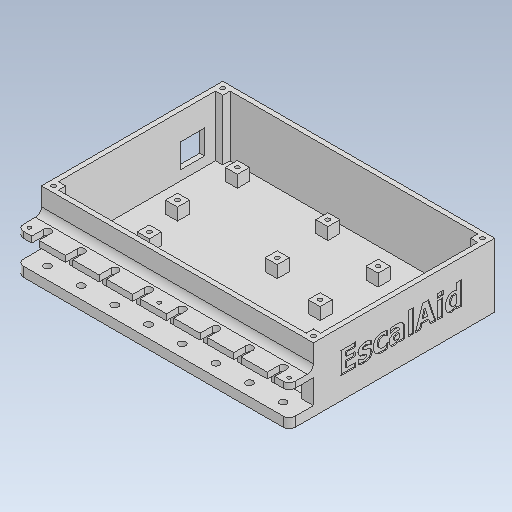
# Autodesk Inventor part: ebox
Saved by Autodesk Inventor 2025.2 (Build 292293000, 293)
## iProperties
Created: 2025-01-01
Part Number: ebox
Material: Generic
Document SubType Name: Modeling
Designer: email
Density: 1 g/cm^3
Appearance: Default
Author: email
Autodesk Inventor part; units mm, degrees
ref_plane "YZ Plane" through (0, 0, 0) normal (1, 0, 0) x (0, 1, 0)
ref_plane "XZ Plane" through (0, 0, 0) normal (0, 1, 0) x (-1, 0, 0)
sketch "Sketch1" plane through (0, 0, 0) normal (0, 1, 0) x (-1, 0, 0)
  line L0 (0, 0) -> (-225, 0)
  line L1 (-225, 0) -> (-225, -150)
  line L2 (-225, -150) -> (0, -150)
  line L3 (0, -150) -> (0, 0)
  line L4 (-12.5, -136.845) -> (-114.1, -136.845)
  line L5 (-114.1, -136.845) -> (-114.1, -83.505)
  line L6 (-114.1, -83.505) -> (-12.5, -83.505)
  line L7 (-12.5, -83.505) -> (-12.5, -136.845)
  line L8 (-4, -4) -> (-221, -4)
  line L9 (-221, -4) -> (-221, -146)
  line L10 (-221, -146) -> (-4, -146)
  line L11 (-4, -146) -> (-4, -4)
  line L12 (-153.3391, -125.2346) -> (-208.3391, -125.2346)
  line L13 (-208.3391, -125.2346) -> (-208.3391, -70.2346)
  line L14 (-208.3391, -70.2346) -> (-153.3391, -70.2346)
  line L15 (-153.3391, -70.2346) -> (-153.3391, -125.2346)
  line L16 (-12.6469, -54.1694) -> (-42.6469, -54.1694)
  line L17 (-42.6469, -54.1694) -> (-42.6469, -34.1694)
  line L18 (-42.6469, -34.1694) -> (-12.6469, -34.1694)
  line L19 (-12.6469, -34.1694) -> (-12.6469, -54.1694)
  line L20 (-15.41, -128.945) -> (-4, -128.945)
  line L21 (-4, -128.945) -> (-4, -117.045)
  line L22 (-4, -117.045) -> (-15.41, -117.045)
  line L23 (-15.41, -117.045) -> (-15.41, -128.945)
  circle A0 centre (-27.74, -134.305) radius 1.75
  circle A1 centre (-26.47, -86.045) radius 1.75
  circle A2 centre (-102.67, -134.305) radius 1.75
  circle A3 centre (-109.02, -86.045) radius 1.75
  circle A4 centre (-156.8391, -121.7346) radius 1.75
  circle A5 centre (-204.8391, -121.7346) radius 1.75
  circle A6 centre (-156.8391, -73.7346) radius 1.75
  circle A7 centre (-204.8391, -73.7346) radius 1.75
  circle A8 centre (-37.5669, -51.6294) radius 1.75
  circle A9 centre (-37.5669, -36.7094) radius 1.75
  line L24 (-22.74, -139.305) -> (-32.74, -139.305)
  line L25 (-32.74, -139.305) -> (-32.74, -129.305)
  line L26 (-32.74, -129.305) -> (-22.74, -129.305)
  line L27 (-22.74, -129.305) -> (-22.74, -139.305)
  line L28 (-22.74, -139.305) -> (-32.74, -129.305) construction
  line L29 (-32.74, -139.305) -> (-22.74, -129.305) construction
  line L30 (-21.47, -81.045) -> (-31.47, -81.045)
  line L31 (-31.47, -81.045) -> (-31.47, -91.045)
  line L32 (-31.47, -91.045) -> (-21.47, -91.045)
  line L33 (-21.47, -91.045) -> (-21.47, -81.045)
  line L34 (-21.47, -81.045) -> (-31.47, -91.045) construction
  line L35 (-31.47, -81.045) -> (-21.47, -91.045) construction
  line L36 (-114.02, -81.045) -> (-104.02, -81.045)
  line L37 (-104.02, -81.045) -> (-104.02, -91.045)
  line L38 (-104.02, -91.045) -> (-114.02, -91.045)
  line L39 (-114.02, -91.045) -> (-114.02, -81.045)
  line L40 (-114.02, -81.045) -> (-104.02, -91.045) construction
  line L41 (-104.02, -81.045) -> (-114.02, -91.045) construction
  line L42 (-107.67, -139.305) -> (-97.67, -139.305)
  line L43 (-97.67, -139.305) -> (-97.67, -129.305)
  line L44 (-97.67, -129.305) -> (-107.67, -129.305)
  line L45 (-107.67, -129.305) -> (-107.67, -139.305)
  line L46 (-107.67, -139.305) -> (-97.67, -129.305) construction
  line L47 (-97.67, -139.305) -> (-107.67, -129.305) construction
  line L48 (-151.8391, -126.7346) -> (-161.8391, -126.7346)
  line L49 (-161.8391, -126.7346) -> (-161.8391, -116.7346)
  line L50 (-161.8391, -116.7346) -> (-151.8391, -116.7346)
  line L51 (-151.8391, -116.7346) -> (-151.8391, -126.7346)
  line L52 (-151.8391, -126.7346) -> (-161.8391, -116.7346) construction
  line L53 (-161.8391, -126.7346) -> (-151.8391, -116.7346) construction
  line L54 (-209.8391, -126.7346) -> (-199.8391, -126.7346)
  line L55 (-199.8391, -126.7346) -> (-199.8391, -116.7346)
  line L56 (-199.8391, -116.7346) -> (-209.8391, -116.7346)
  line L57 (-209.8391, -116.7346) -> (-209.8391, -126.7346)
  line L58 (-209.8391, -126.7346) -> (-199.8391, -116.7346) construction
  line L59 (-199.8391, -126.7346) -> (-209.8391, -116.7346) construction
  line L60 (-209.8391, -68.7346) -> (-199.8391, -68.7346)
  line L61 (-199.8391, -68.7346) -> (-199.8391, -78.7346)
  line L62 (-199.8391, -78.7346) -> (-209.8391, -78.7346)
  line L63 (-209.8391, -78.7346) -> (-209.8391, -68.7346)
  line L64 (-209.8391, -68.7346) -> (-199.8391, -78.7346) construction
  line L65 (-199.8391, -68.7346) -> (-209.8391, -78.7346) construction
  line L66 (-161.8391, -68.7346) -> (-151.8391, -68.7346)
  line L67 (-151.8391, -68.7346) -> (-151.8391, -78.7346)
  line L68 (-151.8391, -78.7346) -> (-161.8391, -78.7346)
  line L69 (-161.8391, -78.7346) -> (-161.8391, -68.7346)
  line L70 (-161.8391, -68.7346) -> (-151.8391, -78.7346) construction
  line L71 (-151.8391, -68.7346) -> (-161.8391, -78.7346) construction
  line L72 (-42.5669, -46.6294) -> (-32.5669, -46.6294)
  line L73 (-32.5669, -46.6294) -> (-32.5669, -56.6294)
  line L74 (-32.5669, -56.6294) -> (-42.5669, -56.6294)
  line L75 (-42.5669, -56.6294) -> (-42.5669, -46.6294)
  line L76 (-42.5669, -46.6294) -> (-32.5669, -56.6294) construction
  line L77 (-32.5669, -46.6294) -> (-42.5669, -56.6294) construction
  line L78 (-32.5669, -41.7094) -> (-42.5669, -41.7094)
  line L79 (-42.5669, -41.7094) -> (-42.5669, -31.7094)
  line L80 (-42.5669, -31.7094) -> (-32.5669, -31.7094)
  line L81 (-32.5669, -31.7094) -> (-32.5669, -41.7094)
  line L82 (-32.5669, -41.7094) -> (-42.5669, -31.7094) construction
  line L83 (-42.5669, -41.7094) -> (-32.5669, -31.7094) construction
  line L84 (0, -4) -> (-225, -4)
  line L85 (-225, -4) -> (-225, 20)
  line L86 (-225, 20) -> (0, 20)
  line L87 (0, 20) -> (0, -4)
  circle A10 centre (-15, 10) radius 2.95
  circle A11 centre (-42.85, 10) radius 2.95
  circle A12 centre (-70.7, 10) radius 2.95
  circle A13 centre (-98.55, 10) radius 2.95
  circle A14 centre (-126.4, 10) radius 2.95
  circle A15 centre (-154.25, 10) radius 2.95
  circle A16 centre (-182.1, 10) radius 2.95
  circle A17 centre (-209.95, 10) radius 2.95
  point P0 (-156.8391, -73.7346)
  point P1 (-225, 8)
  dimension "d0" = 225
  dimension "d1" = 150
  dimension "d2" = 101.6
  dimension "d3" = 53.34
  dimension "d5" = 4
  dimension "d6" = 217
  dimension "d7" = 142
  dimension "d8" = 4
  dimension "d9" = 8.5
  dimension "d10" = 55
  dimension "d11" = 55
  dimension "d12" = 30
  dimension "d13" = 20
  dimension "d14" = 7.9
  dimension "d15" = 8.5
  dimension "d16" = 11.9
  dimension "d17" = 2.54
  dimension "d18" = 3.5
  dimension "d19" = 15.24
  dimension "d20" = 3.5
  dimension "d21" = 3.5
  dimension "d22" = 3.5
  dimension "d23" = 2.54
  dimension "d24" = 13.97
  dimension "d26" = 2.54
  dimension "d27" = 90.17
  dimension "d28" = 2.54
  dimension "d29" = 96.52
  dimension "d30" = 3.5
  dimension "d31" = 3.5
  dimension "d32" = 3.5
  dimension "d33" = 3.5
  dimension "d34" = 3.5
  dimension "d35" = 3.5
  dimension "d36" = 3.5
  dimension "d38" = 3.5
  dimension "d39" = 3.5
  dimension "d40" = 3.5
  dimension "d41" = 3.5
  dimension "d42" = 3.5
  dimension "d43" = 3.5
  dimension "d44" = 2.54
  dimension "d45" = 5.08
  dimension "d46" = 5.08
  dimension "d47" = 2.54
  dimension "d54" = 10
  dimension "d55" = 10
  dimension "d56" = 10
  dimension "d57" = 10
  dimension "d58" = 10
  dimension "d59" = 10
  dimension "d60" = 10
  dimension "d61" = 10
  dimension "d65" = 10
  dimension "d66" = 10
  dimension "d67" = 10
  dimension "d68" = 10
  dimension "d69" = 10
  dimension "d70" = 10
  dimension "d71" = 10
  dimension "d72" = 10
  dimension "d73" = 10
  dimension "d74" = 10
  dimension "d75" = 10
  constraints: 176 end point, 34 parallel, 22 midpoint, 18 centre point, 18 horizontal, 17 perpendicular, 2 point on line, 14 other
  measures "d0" distance of L1.end L2.end
  measures "d1" distance of L0.end L1.end
  measures "d2" distance of L4.start L4.end
  measures "d3" distance of L4.end L5.end
  measures "d5" distance between parallel lines of L0 L8
  measures "d6" distance of L9.end L10.end
  measures "d7" distance of L8.end L9.end
  measures "d8" distance between parallel lines of L3 L11
  measures "d9" distance between parallel lines of L11 L7
  measures "d10" distance of L12.end L13.end
  measures "d11" distance of L13.end L14.end
  measures "d12" distance of L16.start L16.end
  measures "d13" distance of L16.end L17.end
  measures "d14" distance between parallel lines of L4 L20
  measures "d15" distance between parallel lines of L7 L21
  measures "d16" distance of L22.end L20.start
  measures "d17" distance from line of L4 A0.centre
  measures "d18" diameter of A0
  measures "d19" distance from line of L7 A0.centre
  measures "d20" diameter of A1
  measures "d21" diameter of A3
  measures "d22" diameter of A2
  measures "d23" distance from line of L6 A1.centre
  measures "d24" distance from line of L7 A1.centre
  measures "d26" distance from line of L4 A2.centre
  measures "d27" distance from line of A2.centre L7
  measures "d28" distance from line of L6 A3.centre
  measures "d29" distance from line of L7 A3.centre
  measures "d30" diameter of A4
  measures "d31" diameter of A5
  measures "d32" diameter of A6
  measures "d33" diameter of A7
  measures "d34" distance from line of L12 A4.centre
  measures "d35" distance from line of L15 A4.centre
  measures "d36" distance from line of L14 A6.centre
  measures "d38" distance from line of L13 A7.centre
  measures "d39" distance from line of L14 A7.centre
  measures "d40" distance from line of L13 A5.centre
  measures "d41" distance from line of L12 A5.centre
  measures "d42" diameter of A8
  measures "d43" diameter of A9
  measures "d44" distance from line of L16 A8.centre
  measures "d45" distance from line of L17 A8.centre
  measures "d46" distance from line of L17 A9.centre
  measures "d47" distance from line of L18 A9.centre
  measures "d54" distance of L24.end L25.end
  measures "d55" distance of L25.end L26.end
  measures "d56" distance of L42.end L43.end
  measures "d57" distance of L43.end L44.end
  measures "d58" distance of L31.end L32.end
  measures "d59" distance of L30.end L31.end
  measures "d60" distance of L37.end L38.end
  measures "d61" distance of L36.end L37.end
  measures "d65" distance of L48.end L49.end
  measures "d66" distance of L49.end L50.end
  measures "d67" distance of L54.end L55.end
  measures "d68" distance of L55.end L56.end
  measures "d69" distance of L66.end L67.end
  measures "d70" distance of L66.start L66.end
  measures "d71" distance of L62.end L60.start
  measures "d72" distance of L60.start L60.end
  measures "d73" distance of L73.end L74.end
  measures "d74" distance of L72.end L73.end
  measures "d75" distance of L78.start L78.end
extrude "Extrusion1" add sketch "Sketch1" against normal blind 3 contours L3 L84 L8 L1 L0 | L3 L2 L1 L84 L9 L10 L11 | L11 L22 L7 L6 L33 L30 L31 L37 L36 L39 L5 L4 L45 L42 L43 L25 L24 L27 L20 L10 L9 L8 | L11 L20 L7 L22 | L22 L23 L20 L7 L4 L27 L26 L25 L43 L44 L45 L5 L6 L39 L38 L37 L31 L32 L33 | L7 L20 L23 L22 | L33 L32 L31 L6 | L6 L31 L30 L33 | L27 L24 L25 L4 | L4 L25 L26 L27 | L37 L38 L39 L6 | L6 L39 L36 L37 | L43 L42 L45 L4 | L4 L45 L44 L43 | L15 L50 L51 L48 L49 L12 | L12 L49 L50 L15 | L12 L55 L56 L13 L62 L61 L14 L69 L68 L15 L50 L49 | L55 L54 L57 L56 L13 L12 | L12 L13 L56 L55 | L68 L69 L14 L15 | L15 L14 L69 L66 L67 L68 | L62 L63 L60 L61 L14 L13 | L13 L14 L61 L62 | L16 L73 L72 L75 L17 L18 L79 L78 L81 L19 | L73 L74 L75 L16 | L16 L75 L72 L73 | L81 L78 L79 L18 | L18 L79 L80 L81 | A0 | A1 | A2 | A3 | A4 | A5 | A6 | A7 | A8 | A9
extrude "Extrusion2" add sketch "Sketch1" along normal blind 50 contours L3 L84 L8 L1 L0 | L3 L2 L1 L84 L9 L10 L11
extrude "Extrusion3" add sketch "Sketch1" along normal blind 10 contours L33 L32 L31 L6 | L6 L31 L30 L33 | L27 L24 L25 L4 | L4 L25 L26 L27 | L37 L38 L39 L6 | L6 L39 L36 L37 | L43 L42 L45 L4 | L4 L45 L44 L43 | L15 L50 L51 L48 L49 L12 | L12 L49 L50 L15 | L55 L54 L57 L56 L13 L12 | L12 L13 L56 L55 | L68 L69 L14 L15 | L15 L14 L69 L66 L67 L68 | L62 L63 L60 L61 L14 L13 | L13 L14 L61 L62 | L73 L74 L75 L16 | L16 L75 L72 L73 | L81 L78 L79 L18 | L18 L79 L80 L81
extrude "Extrusion4" add sketch "Sketch1" along normal blind 5 and the other way blind 3 contours L0 L85 L86 L87
sketch "Sketch2" plane through (0, 50, 0) normal (0, 0, 1) x (1, 0, 0)
  line L0 (7, -25) -> (23, -25)
  line L1 (23, -25) -> (23, -45)
  line L2 (23, -45) -> (7, -45)
  line L3 (7, -45) -> (7, -25)
  line L4 (7, -25) -> (23, -45) construction
  line L5 (23, -25) -> (7, -45) construction
  line L6 (34.85, -25) -> (50.85, -25)
  line L7 (50.85, -25) -> (50.85, -45)
  line L8 (50.85, -45) -> (34.85, -45)
  line L9 (34.85, -45) -> (34.85, -25)
  line L10 (34.85, -25) -> (50.85, -45) construction
  line L11 (50.85, -25) -> (34.85, -45) construction
  line L12 (62.7, -25) -> (78.7, -25)
  line L13 (78.7, -25) -> (78.7, -45)
  line L14 (78.7, -45) -> (62.7, -45)
  line L15 (62.7, -45) -> (62.7, -25)
  line L16 (62.7, -25) -> (78.7, -45) construction
  line L17 (78.7, -25) -> (62.7, -45) construction
  line L18 (90.55, -25) -> (106.55, -25)
  line L19 (106.55, -25) -> (106.55, -45)
  line L20 (106.55, -45) -> (90.55, -45)
  line L21 (90.55, -45) -> (90.55, -25)
  line L22 (90.55, -25) -> (106.55, -45) construction
  line L23 (106.55, -25) -> (90.55, -45) construction
  line L24 (118.4, -25) -> (134.4, -25)
  line L25 (134.4, -25) -> (134.4, -45)
  line L26 (134.4, -45) -> (118.4, -45)
  line L27 (118.4, -45) -> (118.4, -25)
  line L28 (118.4, -25) -> (134.4, -45) construction
  line L29 (134.4, -25) -> (118.4, -45) construction
  line L30 (146.25, -25) -> (162.25, -25)
  line L31 (162.25, -25) -> (162.25, -45)
  line L32 (162.25, -45) -> (146.25, -45)
  line L33 (146.25, -45) -> (146.25, -25)
  line L34 (146.25, -25) -> (162.25, -45) construction
  line L35 (162.25, -25) -> (146.25, -45) construction
  line L36 (174.1, -25) -> (190.1, -25)
  line L37 (190.1, -25) -> (190.1, -45)
  line L38 (190.1, -45) -> (174.1, -45)
  line L39 (174.1, -45) -> (174.1, -25)
  line L40 (174.1, -25) -> (190.1, -45) construction
  line L41 (190.1, -25) -> (174.1, -45) construction
  line L42 (201.95, -25) -> (217.95, -25)
  line L43 (217.95, -25) -> (217.95, -45)
  line L44 (217.95, -45) -> (201.95, -45)
  line L45 (201.95, -45) -> (201.95, -25)
  line L46 (201.95, -25) -> (217.95, -45) construction
  line L47 (217.95, -25) -> (201.95, -45) construction
  line L48 (0, -45) -> (0, 0) projected
  line L49 (0, -45) -> (225, -45) projected
  point P0 (15, -35)
  point P1 (42.85, -35)
  point P2 (70.7, -35)
  point P3 (98.55, -35)
  point P4 (126.4, -35)
  point P5 (154.25, -35)
  point P6 (182.1, -35)
  point P7 (209.95, -35)
  dimension "d105" = 16
  dimension "d106" = 20
  dimension "d109" = 27.85
  dimension "d132" = 15
  dimension "d133" = 10
  constraints: 96 end point, 16 midpoint, 2 horizontal, 2 parallel, 1 collinear, 1 perpendicular, 76 other
  measures "d105" distance of L0.start L0.end
  measures "d106" distance of L2.end L0.start
  measures "d109" distance of L0.start L6.start
  measures "d132" distance from line of L48 point (15, -35)
  measures "d133" distance from line of L49 point (15, -35)
extrude "Extrusion5" cut sketch "Sketch2" against normal blind 4
ref_plane "Work Plane1" through (0, 25, 0) normal (0, 1, 0) x (1, 0, 0)
sketch "Sketch3" plane through (0, 25, 0) normal (0, 1, 0) x (1, 0, 0)
  line L0 (0, 150) -> (0, 0) projected
  line L1 (0, 0) -> (225, 0)
  line L2 (225, 0) -> (225, -20)
  line L3 (225, -20) -> (0, -20)
  line L4 (0, -20) -> (0, 0)
  circle A0 centre (15, -10) radius 2.95 construction
  line L5 (11.95, -10) -> (11.95, -20)
  line L6 (18.05, -9.9879) -> (18.05, -20)
  arc A1 (18.05, -9.9879) -> (11.95, -10) centre (15, -10) ccw
  line L7 (11.95, -20) -> (18.05, -20)
  line L8 (39.8, -10) -> (39.8, -20)
  line L9 (45.9, -9.9879) -> (45.9, -20)
  arc A2 (45.9, -9.9879) -> (39.8, -10) centre (42.85, -10) ccw
  line L10 (39.8, -20) -> (45.9, -20)
  line L11 (67.65, -10) -> (67.65, -20)
  line L12 (73.75, -9.9879) -> (73.75, -20)
  arc A3 (73.75, -9.9879) -> (67.65, -10) centre (70.7, -10) ccw
  line L13 (67.65, -20) -> (73.75, -20)
  line L14 (95.5, -10) -> (95.5, -20)
  line L15 (101.6, -9.9879) -> (101.6, -20)
  arc A4 (101.6, -9.9879) -> (95.5, -10) centre (98.55, -10) ccw
  line L16 (95.5, -20) -> (101.6, -20)
  line L17 (123.35, -10) -> (123.35, -20)
  line L18 (129.45, -9.9879) -> (129.45, -20)
  arc A5 (129.45, -9.9879) -> (123.35, -10) centre (126.4, -10) ccw
  line L19 (123.35, -20) -> (129.45, -20)
  line L20 (151.2, -10) -> (151.2, -20)
  line L21 (157.3, -9.9879) -> (157.3, -20)
  arc A6 (157.3, -9.9879) -> (151.2, -10) centre (154.25, -10) ccw
  line L22 (151.2, -20) -> (157.3, -20)
  line L23 (179.05, -10) -> (179.05, -20)
  line L24 (185.15, -9.9879) -> (185.15, -20)
  arc A7 (185.15, -9.9879) -> (179.05, -10) centre (182.1, -10) ccw
  line L25 (179.05, -20) -> (185.15, -20)
  line L26 (206.9, -10) -> (206.9, -20)
  line L27 (213, -9.9879) -> (213, -20)
  arc A8 (213, -9.9879) -> (206.9, -10) centre (209.95, -10) ccw
  line L28 (206.9, -20) -> (213, -20)
  circle A9 centre (5, -15) radius 1.5
  circle A10 centre (220, -15) radius 1.5
  circle A11 centre (112.5, -15) radius 1.5
  point P0 (18.125, -20)
  point P1 (45.975, -20)
  point P2 (73.825, -20)
  point P3 (101.675, -20)
  point P4 (129.525, -20)
  point P5 (157.375, -20)
  point P6 (185.225, -20)
  point P7 (213.075, -20)
  point P8 (112.5, -20)
  dimension "d118" = 20
  dimension "d119" = 225
  dimension "d140" = 27.85
  dimension "d145" = 3.05
  dimension "d146" = 3
  dimension "d147" = 5
  dimension "d148" = 5
  dimension "d149" = 3
  dimension "d150" = 5
  dimension "d151" = 5
  dimension "d152" = 3
  dimension "d153" = 5
  constraints: 54 end point, 49 horizontal alignment, 16 point on circle, 15 parallel, 11 centre point, 7 collinear, 7 equal radius, 3 horizontal, 2 vertical, 1 coincident, 1 perpendicular, 1 tangent, 7 other
  measures "d118" distance of L1.end L2.end
  measures "d119" distance of L2.end L4.start
  measures "d140" distance of A0.centre point (42.85, -10)
  measures "d145" radius of A1
  measures "d146" diameter of A9
  measures "d147" distance from line of L4 A9.centre
  measures "d149" diameter of A10
  measures "d150" distance from line of L2 A10.centre
  measures "d152" diameter of A11
  measures "d153" distance of point (112.5, -20) A11.centre
extrude "Extrusion6" add sketch "Sketch3" along normal blind 5 contours L1 L2 L3 L27 A8 L26 L24 A7 L23 L21 A6 L20 L18 A5 L17 L15 A4 L14 L12 A3 L11 L9 A2 L8 L6 A1 L5 L4
fillet "Fillet2" radius 5 4 edges at (0, 27.5, 20) (0, 1, 20) (225, 27.5, 20) (225, 1, 20)
fillet "Fillet3" radius 5 1 edges at (112.5, 30, 0)
sketch "Sketch4" plane through (0, 50, 0) normal (0, 1, 0) x (1, 0, 0)
  line L0 (0, 0) -> (10, 0)
  line L1 (10, 0) -> (10, 10)
  line L2 (10, 10) -> (0, 10)
  line L3 (0, 10) -> (0, 0)
  circle A0 centre (5, 5) radius 1.75
  line L4 (0, -15) -> (0, 150) projected
  line L5 (0, 150) -> (10, 150)
  line L6 (10, 150) -> (10, 140)
  line L7 (10, 140) -> (0, 140)
  line L8 (0, 140) -> (0, 150)
  circle A1 centre (5, 145) radius 1.75
  line L9 (0, 150) -> (225, 150) projected
  line L10 (225, 150) -> (215, 150)
  line L11 (215, 150) -> (215, 140)
  line L12 (215, 140) -> (225, 140)
  line L13 (225, 140) -> (225, 150)
  line L14 (7, 0) -> (23, 0) projected
  line L15 (225, 0) -> (215, 0)
  line L16 (215, 0) -> (215, 10)
  line L17 (215, 10) -> (225, 10)
  line L18 (225, 10) -> (225, 0)
  circle A2 centre (220, 145) radius 1.75
  circle A3 centre (220, 5) radius 1.75
  point P0 (5, 10)
  point P1 (5, 140)
  point P2 (10, 145)
  point P3 (217.95, 0)
  point P4 (215, 145)
  point P5 (220, 140)
  point P6 (217.95, 0)
  point P7 (215, 5)
  dimension "d154" = 10
  dimension "d155" = 10
  dimension "d156" = 3.5
  dimension "d157" = 5
  dimension "d158" = 5
  dimension "d159" = 10
  dimension "d160" = 10
  dimension "d161" = 3.5
  dimension "d162" = 5
  dimension "d163" = 5
  dimension "d164" = 10
  dimension "d165" = 10
  dimension "d166" = 3.5
  dimension "d167" = 5
  dimension "d168" = 5
  dimension "d169" = 10
  dimension "d170" = 10
  dimension "d171" = 3.5
  dimension "d182" = 5
  dimension "d183" = 5
  constraints: 32 end point, 11 equal length, 6 midpoint, 4 centre point, 4 horizontal, 4 perpendicular
  measures "d154" distance of L1.end L2.end
  measures "d155" distance of L0.end L1.end
  measures "d156" diameter of A0
  measures "d157" distance of point (5, 10) A0.centre
  measures "d158" distance from line of L1 A0.centre
  measures "d159" distance of L5.end L6.end
  measures "d160" distance of L6.end L7.end
  measures "d161" diameter of A1
  measures "d162" distance of point (5, 140) A1.centre
  measures "d163" distance of point (10, 145) A1.centre
  measures "d164" distance of L10.end L11.end
  measures "d165" distance of L11.end L12.end
  measures "d166" diameter of A2
  measures "d167" distance of point (215, 145) A2.centre
  measures "d168" distance of point (220, 140) A2.centre
  measures "d169" distance of L16.end L17.end
  measures "d170" distance of L15.end L16.end
  measures "d171" diameter of A3
  measures "d182" distance from line of L17 A3.centre
  measures "d183" distance of point (215, 5) A3.centre
extrude "Extrusion7" add sketch "Sketch4" against normal up to surface (50 mm away) contours L3 L2 L1 L0 | L9 L13 L12 L11 | L4 L5 L6 L7 | A0 | A1 | L15 L16 L17 L18 | A2 | A3
extrude "Extrusion8" cut sketch "Sketch4" against normal blind 10 contours A0 | A1 | A2 | A3
sketch "Sketch5" plane through (0, -3, -150) normal (-1, 0, 0) x (0, 0, 1)
  line L0 (19, 31) -> (39, 31)
  line L1 (39, 31) -> (39, 11)
  line L2 (39, 11) -> (19, 11)
  line L3 (19, 11) -> (19, 31)
  line L4 (10, 3) -> (140, 3) projected
  line L5 (4, 3) -> (4, 43)
  point P0 (150, 3)
  dimension "d176" = 20
  dimension "d177" = 20
  dimension "d180" = 8
  dimension "d181" = 15
  constraints: 10 end point, 2 parallel, 1 horizontal, 1 perpendicular
  measures "d176" distance of L0.start L0.end
  measures "d177" distance of L2.end L0.start
  measures "d180" distance between parallel lines of L4 L2
  measures "d181" distance between parallel lines of L5 L3
extrude "Extrusion9" cut sketch "Sketch5" against normal up to surface (4 mm away)
sketch "Sketch6" plane through (225, -3, -150) normal (1, 0, 0) x (0, 0, -1)
  line L0 (-128.9736, 36.905) -> (-79.4193, 36.905) construction
  line L1 (-79.4193, 36.905) -> (-79.4193, 26.2486) construction
  line L2 (-79.4193, 26.2486) -> (-128.9736, 26.2486) construction
  line L3 (-128.9736, 26.2486) -> (-128.9736, 36.905) construction
  line L4 (-127.1065, 18.0882) -> (-127.1065, 36.0882)
  line L5 (-127.1065, 36.0882) -> (-114.9412, 36.0882)
  line L6 (-114.9412, 36.0882) -> (-114.9412, 32.6603)
  line L7 (-114.9412, 32.6603) -> (-122.6138, 32.6603)
  line L8 (-122.6138, 32.6603) -> (-122.6138, 29.495)
  line L9 (-122.6138, 29.495) -> (-115.5393, 29.495)
  line L10 (-115.5393, 29.495) -> (-115.5393, 26.0671)
  line L11 (-115.5393, 26.0671) -> (-122.6138, 26.0671)
  line L12 (-122.6138, 26.0671) -> (-122.6138, 21.516)
  line L13 (-122.6138, 21.516) -> (-114.9412, 21.516)
  line L14 (-114.9412, 21.516) -> (-114.9412, 18.0882)
  line L15 (-114.9412, 18.0882) -> (-127.1065, 18.0882)
  spline S0 degree 2 poles (-107.9979, 17.7235) (-109.4858, 17.7235) (-112.1552, 18.3799) (-113.0304, 18.8175) knots 0 0 0 1 2 2 2
  line L16 (-113.0304, 18.8175) -> (-113.0304, 22.3912)
  line L17 (-113.0304, 22.3912) -> (-112.6803, 22.3912)
  spline S1 degree 2 poles (-112.6803, 22.3912) (-112.374, 22.1579) (-111.6009, 21.6036) (-110.9153, 21.2972) knots 0 0 0 1 2 2 2
  spline S2 degree 2 poles (-110.9153, 21.2972) (-110.3172, 21.0201) (-108.844, 20.6262) (-107.9688, 20.6262) knots 0 0 0 1 2 2 2
  spline S3 degree 2 poles (-107.9688, 20.6262) (-107.079, 20.6262) (-105.7078, 21.1805) (-105.7078, 21.7786) knots 0 0 0 1 2 2 2
  spline S4 degree 2 poles (-105.7078, 21.7786) (-105.7078, 22.2454) (-106.3351, 22.7413) (-107.2394, 22.9455) knots 0 0 0 1 2 2 2
  spline S5 degree 2 poles (-107.2394, 22.9455) (-107.7208, 23.0768) (-109.1941, 23.354) (-109.7629, 23.529) knots 0 0 0 1 2 2 2
  spline S6 degree 2 poles (-109.7629, 23.529) (-111.3675, 24.025) (-112.972, 25.965) (-112.972, 27.5549) knots 0 0 0 1 2 2 2
  spline S7 degree 2 poles (-112.972, 27.5549) (-112.972, 28.4593) (-112.1406, 30.0639) (-111.3237, 30.6911) knots 0 0 0 1 2 2 2
  spline S8 degree 2 poles (-111.3237, 30.6911) (-110.5214, 31.3037) (-108.1438, 32.0331) (-106.6414, 32.0331) knots 0 0 0 1 2 2 2
  spline S9 degree 2 poles (-106.6414, 32.0331) (-105.2119, 32.0331) (-102.8197, 31.4642) (-102.0028, 31.0703) knots 0 0 0 1 2 2 2
  line L18 (-102.0028, 31.0703) -> (-102.0028, 27.6279)
  line L19 (-102.0028, 27.6279) -> (-102.3383, 27.6279)
  spline S10 degree 2 poles (-102.3383, 27.6279) (-102.5571, 27.8029) (-103.5052, 28.3718) (-103.9428, 28.576) knots 0 0 0 1 2 2 2
  spline S11 degree 2 poles (-103.9428, 28.576) (-104.4825, 28.8094) (-105.7953, 29.1303) (-106.4809, 29.1303) knots 0 0 0 1 2 2 2
  spline S12 degree 2 poles (-106.4809, 29.1303) (-107.3999, 29.1303) (-108.6689, 28.5031) (-108.6689, 27.9925) knots 0 0 0 1 2 2 2
  spline S13 degree 2 poles (-108.6689, 27.9925) (-108.6689, 27.5258) (-108.0417, 27.0006) (-106.9915, 26.7381) knots 0 0 0 1 2 2 2
  spline S14 degree 2 poles (-106.9915, 26.7381) (-106.4518, 26.6068) (-105.0368, 26.3588) (-104.3804, 26.14) knots 0 0 0 1 2 2 2
  spline S15 degree 2 poles (-104.3804, 26.14) (-102.9218, 25.6733) (-101.4047, 23.8499) (-101.4047, 22.3329) knots 0 0 0 1 2 2 2
  spline S16 degree 2 poles (-101.4047, 22.3329) (-101.4047, 21.3848) (-102.2945, 19.6489) (-103.126, 19.0655) knots 0 0 0 1 2 2 2
  spline S17 degree 2 poles (-103.126, 19.0655) (-103.9866, 18.4237) (-106.3496, 17.7235) (-107.9979, 17.7235) knots 0 0 0 1 2 2 2
  spline S18 degree 2 poles (-92.7402, 17.7235) (-94.4177, 17.7235) (-97.2038, 18.5695) (-98.2394, 19.4447) knots 0 0 0 1 2 2 2
  spline S19 degree 2 poles (-98.2394, 19.4447) (-99.2459, 20.3345) (-100.3837, 23.0039) (-100.3837, 24.8126) knots 0 0 0 1 2 2 2
  spline S20 degree 2 poles (-100.3837, 24.8126) (-100.3837, 26.7673) (-99.1584, 29.495) (-98.0936, 30.3702) knots 0 0 0 1 2 2 2
  spline S21 degree 2 poles (-98.0936, 30.3702) (-97.0871, 31.2162) (-94.3448, 32.0331) (-92.8569, 32.0331) knots 0 0 0 1 2 2 2
  spline S22 degree 2 poles (-92.8569, 32.0331) (-91.7338, 32.0331) (-89.4874, 31.5079) (-88.3496, 30.9391) knots 0 0 0 1 2 2 2
  line L20 (-88.3496, 30.9391) -> (-88.3496, 27.3215)
  line L21 (-88.3496, 27.3215) -> (-88.8894, 27.3215)
  spline S23 degree 2 poles (-88.8894, 27.3215) (-89.1519, 27.5695) (-89.8812, 28.153) (-90.3188, 28.3864) knots 0 0 0 1 2 2 2
  spline S24 degree 2 poles (-90.3188, 28.3864) (-90.7856, 28.6489) (-91.938, 28.999) (-92.6527, 28.999) knots 0 0 0 1 2 2 2
  spline S25 degree 2 poles (-92.6527, 28.999) (-94.2718, 28.999) (-96.0514, 26.7381) (-96.0514, 24.8126) knots 0 0 0 1 2 2 2
  spline S26 degree 2 poles (-96.0514, 24.8126) (-96.0514, 22.7705) (-94.1552, 20.7575) (-92.5798, 20.7575) knots 0 0 0 1 2 2 2
  spline S27 degree 2 poles (-92.5798, 20.7575) (-91.7775, 20.7575) (-90.5814, 21.1222) (-90.1438, 21.3848) knots 0 0 0 1 2 2 2
  spline S28 degree 2 poles (-90.1438, 21.3848) (-89.7208, 21.6327) (-89.1082, 22.187) (-88.8894, 22.4058) knots 0 0 0 1 2 2 2
  line L22 (-88.8894, 22.4058) -> (-88.3496, 22.4058)
  line L23 (-88.3496, 22.4058) -> (-88.3496, 18.7737)
  spline S29 degree 2 poles (-88.3496, 18.7737) (-88.7143, 18.6133) (-89.6624, 18.2049) (-90.1584, 18.0736) knots 0 0 0 1 2 2 2
  spline S30 degree 2 poles (-90.1584, 18.0736) (-90.771, 17.8985) (-91.8505, 17.7235) (-92.7402, 17.7235) knots 0 0 0 1 2 2 2
  spline S31 degree 2 poles (-78.8537, 19.5322) (-79.2913, 19.1676) (-79.9769, 18.5841) (-80.5603, 18.2924) knots 0 0 0 1 2 2 2
  spline S32 degree 2 poles (-80.5603, 18.2924) (-81.1292, 18.0152) (-82.2086, 17.7235) (-83.1714, 17.7235) knots 0 0 0 1 2 2 2
  spline S33 degree 2 poles (-83.1714, 17.7235) (-84.9801, 17.7235) (-87.3577, 20.1449) (-87.3577, 21.9828) knots 0 0 0 1 2 2 2
  spline S34 degree 2 poles (-87.3577, 21.9828) (-87.3577, 23.4852) (-86.1471, 25.3523) (-85.0093, 25.8921) knots 0 0 0 1 2 2 2
  spline S35 degree 2 poles (-85.0093, 25.8921) (-83.8569, 26.4463) (-80.6624, 26.8839) (-78.8245, 27.0006) knots 0 0 0 1 2 2 2
  line L24 (-78.8245, 27.0006) -> (-78.8245, 27.0736)
  spline S36 degree 2 poles (-78.8245, 27.0736) (-78.8245, 28.1968) (-80.4874, 29.0574) (-82.1503, 29.0574) knots 0 0 0 1 2 2 2
  spline S37 degree 2 poles (-82.1503, 29.0574) (-82.8942, 29.0574) (-84.9072, 28.5177) (-85.8553, 28.0946) knots 0 0 0 1 2 2 2
  line L25 (-85.8553, 28.0946) -> (-86.22, 28.0946)
  line L26 (-86.22, 28.0946) -> (-86.22, 31.3767)
  spline S38 degree 2 poles (-86.22, 31.3767) (-85.5928, 31.5517) (-82.7921, 32.0476) (-81.3626, 32.0476) knots 0 0 0 1 2 2 2
  spline S39 degree 2 poles (-81.3626, 32.0476) (-77.8618, 32.0476) (-74.6527, 29.7138) (-74.6527, 27.3215) knots 0 0 0 1 2 2 2
  line L27 (-74.6527, 27.3215) -> (-74.6527, 18.0882)
  line L28 (-74.6527, 18.0882) -> (-78.8537, 18.0882)
  line L29 (-78.8537, 18.0882) -> (-78.8537, 19.5322)
  line L30 (-78.8537, 21.6327) -> (-78.8537, 24.448)
  spline S40 degree 2 poles (-78.8537, 24.448) (-79.9331, 24.3459) (-81.2605, 24.1854) (-81.9023, 23.952) knots 0 0 0 1 2 2 2
  spline S41 degree 2 poles (-81.9023, 23.952) (-82.4712, 23.7624) (-83.0838, 22.9747) (-83.0838, 22.3329) knots 0 0 0 1 2 2 2
  spline S42 degree 2 poles (-83.0838, 22.3329) (-83.0838, 21.3848) (-82.0482, 20.67) (-81.0417, 20.67) knots 0 0 0 1 2 2 2
  spline S43 degree 2 poles (-81.0417, 20.67) (-80.4874, 20.67) (-79.3205, 21.1805) (-78.8537, 21.6327) knots 0 0 0 1 2 2 2
  line L31 (-67.2864, 18.0882) -> (-71.5166, 18.0882)
  line L32 (-71.5166, 18.0882) -> (-71.5166, 36.8904)
  line L33 (-71.5166, 36.8904) -> (-67.2864, 36.8904)
  line L34 (-67.2864, 36.8904) -> (-67.2864, 18.0882)
  line L35 (-65.7402, 18.0882) -> (-59.6576, 36.0882)
  line L36 (-59.6576, 36.0882) -> (-54.7273, 36.0882)
  line L37 (-54.7273, 36.0882) -> (-48.6446, 18.0882)
  line L38 (-48.6446, 18.0882) -> (-53.2978, 18.0882)
  line L39 (-53.2978, 18.0882) -> (-54.421, 21.764)
  line L40 (-54.421, 21.764) -> (-60.0806, 21.764)
  line L41 (-60.0806, 21.764) -> (-61.2184, 18.0882)
  line L42 (-61.2184, 18.0882) -> (-65.7402, 18.0882)
  line L43 (-55.4129, 25.0314) -> (-57.2508, 30.9828)
  line L44 (-57.2508, 30.9828) -> (-59.1033, 25.0314)
  line L45 (-59.1033, 25.0314) -> (-55.4129, 25.0314)
  line L46 (-42.8683, 18.0882) -> (-47.0984, 18.0882)
  line L47 (-47.0984, 18.0882) -> (-47.0984, 31.6684)
  line L48 (-47.0984, 31.6684) -> (-42.8683, 31.6684)
  line L49 (-42.8683, 31.6684) -> (-42.8683, 18.0882)
  line L50 (-42.737, 33.6084) -> (-47.2151, 33.6084)
  line L51 (-47.2151, 33.6084) -> (-47.2151, 36.905)
  line L52 (-47.2151, 36.905) -> (-42.737, 36.905)
  line L53 (-42.737, 36.905) -> (-42.737, 33.6084)
  line L54 (-27.2897, 18.0882) -> (-31.5198, 18.0882)
  line L55 (-31.5198, 18.0882) -> (-31.5198, 19.5031)
  spline S44 degree 2 poles (-31.5198, 19.5031) (-31.9283, 19.1676) (-32.9785, 18.3945) (-33.3869, 18.1903) knots 0 0 0 1 2 2 2
  spline S45 degree 2 poles (-33.3869, 18.1903) (-33.8829, 17.9569) (-34.8748, 17.7089) (-35.5603, 17.7089) knots 0 0 0 1 2 2 2
  spline S46 degree 2 poles (-35.5603, 17.7089) (-37.8796, 17.7089) (-40.5928, 21.5598) (-40.5928, 24.7689) knots 0 0 0 1 2 2 2
  spline S47 degree 2 poles (-40.5928, 24.7689) (-40.5928, 26.5485) (-39.6738, 29.1595) (-38.8715, 30.1222) knots 0 0 0 1 2 2 2
  spline S48 degree 2 poles (-38.8715, 30.1222) (-38.1276, 31.012) (-36.0271, 32.0331) (-34.8602, 32.0331) knots 0 0 0 1 2 2 2
  spline S49 degree 2 poles (-34.8602, 32.0331) (-33.7954, 32.0331) (-32.4242, 31.5809) (-31.5198, 31.1141) knots 0 0 0 1 2 2 2
  line L56 (-31.5198, 31.1141) -> (-31.5198, 36.8904)
  line L57 (-31.5198, 36.8904) -> (-27.2897, 36.8904)
  line L58 (-27.2897, 36.8904) -> (-27.2897, 18.0882)
  line L59 (-31.5198, 21.8224) -> (-31.5198, 28.4885)
  spline S50 degree 2 poles (-31.5198, 28.4885) (-31.8261, 28.6489) (-32.8472, 28.8532) (-33.2119, 28.8532) knots 0 0 0 1 2 2 2
  spline S51 degree 2 poles (-33.2119, 28.8532) (-34.7289, 28.8532) (-36.2605, 26.7235) (-36.2605, 24.8126) knots 0 0 0 1 2 2 2
  spline S52 degree 2 poles (-36.2605, 24.8126) (-36.2605, 22.7997) (-35.0352, 21.0055) (-33.6787, 21.0055) knots 0 0 0 1 2 2 2
  spline S53 degree 2 poles (-33.6787, 21.0055) (-33.1244, 21.0055) (-31.9866, 21.4431) (-31.5198, 21.8224) knots 0 0 0 1 2 2 2
  point P0 (-150, 3)
  constraints: 2 other
extrude "Extrusion10" cut sketch "Sketch6" against normal blind 1
body "Solid1"
